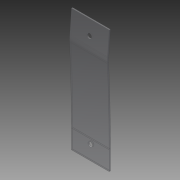
# Autodesk Inventor part: Hopper to Pail Polycarbonate Flap Connector V2
Saved by Autodesk Inventor 2014 SP1 (Build 180222100, 222)
## iProperties
Created: 2013-12-18
Part Number: Hopper to Pail Polycarbonate Flap Connector V2
Material: Polycarbonate, Clear
Document SubType Name: Modeling
Designer: Moses
Mass: 1.9834 g
Surface Area: 43.5191 cm^2
Volume: 1.65283 cm^3
Density: 1.2 g/cm^3
Appearance: Polycarbonate - Clear
Author: Moses
Autodesk Inventor part; units mm, degrees
ref_plane "YZ Plane" through (0, 0, 0) normal (1, 0, 0) x (0, 1, 0)
ref_plane "XZ Plane" through (0, 0, 0) normal (0, 1, 0) x (-1, 0, 0)
sketch "Sketch1" plane through (0, 0, 0) normal (0, 0, 1) x (1, 0, 0)
  line L0 (0, 0) -> (25.4, 0)
  line L1 (25.4, 0) -> (25.4, 82.55)
  line L2 (25.4, 82.55) -> (0, 82.55)
  line L3 (0, 82.55) -> (0, 0)
  line L4 (12.7, 82.55) -> (12.7, 0) construction
  circle A0 centre (12.7, 73.025) radius 1.5875
  circle A1 centre (12.7, 9.525) radius 1.5875
  dimension "d0" = 25.4
  dimension "d1" = 82.55
  dimension "d2" = 3.175
  dimension "d3" = 9.525
  dimension "d4" = 9.525
  constraints: 10 end point, 2 centre point, 2 midpoint, 2 parallel, 2 point on line, 1 equal radius, 1 horizontal, 1 perpendicular
  measures "d0" distance of L2.end L1.end
  measures "d1" distance of L1.end L0.end
  measures "d2" diameter of A0
  measures "d3" distance from line of L2 A0.centre
  measures "d4" distance from line of L0 A1.centre
extrude "Extrusion1" add sketch "Sketch1" along normal blind 0.7937
ref_plane "Work Plane1" through (12.7, 0, 0) normal (1, 0, 0) x (0, 0, -1)
sketch "Sketch2" plane through (25.4, 0, 0) normal (1, 0, 0) x (0, 0, -1)
  line L0 (0, 0) -> (0, 82.55) projected
  line L1 (0, 82.55) -> (-0.7937, 82.55) projected
  line L2 (-0.7937, 0) -> (-0.7937, 82.55) projected
  line L3 (0, 0) -> (-0.7937, 0) projected
  line L4 (1.093, 107.9388) -> (-6.4365, 6.6182) construction
  line L5 (1.093, 107.9388) -> (127.7437, 98.527) construction
  line L6 (-0.7937, 82.55) -> (-2.2055, 63.5524)
  arc A0 (-2.2055, 63.5524) -> (-2.2278, 60.3774) centre (21.3863, 61.7992) ccw
  line L7 (-0.7937, 0) -> (-0.7937, 12.7)
  arc A1 (-0.7937, 12.7) -> (-2.2278, 60.3774) centre (-794.0664, 12.7) ccw
  line L8 (-0.7937, 82.55) -> (-0.0022, 82.4912)
  line L9 (-0.0022, 82.4912) -> (-1.4139, 63.4936)
  line L10 (-0.7937, 12.7) -> (0, 12.7) construction
  line L11 (-0.7937, 0) -> (0, 0)
  line L12 (0, 12.7) -> (0, 0)
  arc A2 (0, 12.7) -> (-1.4355, 60.4251) centre (-794.0664, 12.7) ccw
  arc A3 (-1.4139, 63.4936) -> (-1.4355, 60.4251) centre (21.3863, 61.7992) ccw
  dimension "d7" = 85.75
  dimension "d8" = 19.05
  dimension "d9" = 12.7
  dimension "d12" = 0.7937
  dimension "d15" = 101.6
  dimension "d16" = 127
  dimension "d17" = 25.4
  dimension "d30" = 3.175
  constraints: 18 end point, 8 point on circle, 4 centre point, 4 point on line, 3 perpendicular, 3 tangent, 2 horizontal, 1 other
  measures "d7" angle of L5 L0
  measures "d8" distance of L1.end L6.end
  measures "d9" distance of L2.start L7.end
  measures "d12" distance of L1.end L8.end
  measures "d15" distance of L4.start L4.end
  measures "d16" distance of L4.start L5.end
  measures "d17" distance from line of L5 L0.end
  measures "d30" vertical distance of A0.end L6.end
extrude "Extrusion2" cut sketch "Sketch2" against normal blind 25.4 contours L3 L2 A2 L0 | A2 L2 L9 L8 L1 L0 | L8 L9 L2
extrude "Extrusion3" add sketch "Sketch2" against normal blind 25.4 contours L3 L2 A2 L0 | L2 A1 A0 L6 L9 A3 A2 | L8 L9 L2
sketch "Sketch3" plane through (25.4, 63.4936, 1.4139) normal (0, -0.0741085, -0.9972502) x (-1, 0, 0)
  line L0 (0, 0) -> (25.4, 0) projected
  line L1 (0, 19.05) -> (25.4, 19.05) projected
  line L2 (12.7, 19.05) -> (12.7, 0) construction
  circle A0 centre (12.7, 9.525) radius 1.5875
  point P0 (25.4, -63.2142)
  dimension "d22" = 3.175
  dimension "d23" = 9.525
  constraints: 3 midpoint, 2 end point, 1 centre point
  measures "d22" diameter of A0
  measures "d23" distance from line of L1 A0.centre
extrude "Extrusion4" cut sketch "Sketch3" against normal through all
sketch "Sketch4" plane through (25.4, 0, 0) normal (0, 0, -1) x (-1, 0, 0)
  line L0 (0, 0) -> (25.4, 0) projected
  line L1 (0, 12.7) -> (25.4, 12.7) projected
  line L2 (12.7, 12.7) -> (12.7, 0) construction
  circle A0 centre (12.7, 9.525) radius 1.5875
  dimension "d26" = 3.175
  dimension "d27" = 9.525
  constraints: 2 end point, 2 midpoint, 1 centre point, 1 point on line
  measures "d26" diameter of A0
  measures "d27" distance of L2.end A0.centre
extrude "Extrusion5" cut sketch "Sketch4" against normal through all
equation "\"d4\" = d3"
equation "\"d12\" = d11"
equation "\"d11\" = 0.79375"
body "Solid1"
